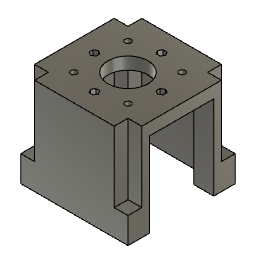
底座第三版v1 v3 (Autodesk Fusion 360 design; units mm, degrees)
Autodesk Fusion 360 part; units mm, degrees
sketch "草图1" plane through (0, 0, 0) normal (0, 0, 1) x (1, 0, 0)
  line L0 (0, 0) -> (70, 0)
  line L1 (70, 0) -> (70, 70)
  line L2 (70, 70) -> (0, 70)
  line L3 (0, 70) -> (0, 0)
  dimension "d1" = 70
  dimension "d2" = 70
  constraint horizontal L0
  constraint vertical L1
  constraint horizontal L2
  constraint vertical L3
  constraint coincident L0.start L3.end
  measures "d1" distance of L0.start L0.end
  measures "d2" distance of L0.start L2.end
extrude "拉伸1" add sketch "草图1" along normal blind 20
sketch "草图2" plane through (0, 0, 20) normal (0, 0, 1) x (-1, 0, 0)
  line L0 (0, -70) -> (0, 0)
  line L1 (0, 0) -> (-70, 0)
  line L2 (-70, 0) -> (-70, -70)
  line L3 (-70, -70) -> (0, -70)
  line L4 (-13.4, -56.6) -> (-56.6, -56.6)
  line L5 (-56.6, -56.6) -> (-56.6, -13.4)
  line L6 (-56.6, -13.4) -> (-13.4, -13.4)
  line L7 (-13.4, -13.4) -> (-13.4, -56.6)
  dimension "d5" = 43.2
  dimension "d6" = 43.2
  dimension "d7" = 13.4
  dimension "d8" = 13.4
  constraint horizontal L4
  constraint vertical L5
  constraint horizontal L6
  constraint vertical L7
  measures "d5" distance of L4.start L4.end
  measures "d6" distance of L4.start L6.end
  measures "d7" distance of L0 L7
  measures "d8" distance of L3 L4
extrude "拉伸2" cut sketch "草图2" against normal blind 6.5 contours L4 L5 L6 L7
sketch "草图3" plane through (0, 0, 13.5) normal (0, 0, 1) x (-1, 0, 0)
  line L0 (-13.4, -13.4) -> (-56.6, -13.4)
  line L1 (-56.6, -13.4) -> (-56.6, -56.6)
  line L2 (-56.6, -56.6) -> (-13.4, -56.6)
  line L3 (-13.4, -56.6) -> (-13.4, -13.4)
  circle A0 centre (-35, -35) radius 25
  line L4 (-56.6, -13.4) -> (-35, -35)
  circle A1 centre (-52.6777, -17.3223) radius 0.4987
  point P0 (-52.6777, -52.6777)
  point P1 (-17.3223, -52.6777)
  point P2 (-17.3223, -17.3223)
  dimension "d11" = 50
  dimension "d12" = 21.6
  dimension "d13" = 21.6
  dimension "d15" = 360
  constraint coincident L0.end L1.start
  constraint coincident A0.centre L4.end
  constraint coincident L4 A1.centre
  constraint coincident A0 A1.centre
  measures "d11" diameter of A0
  measures "d12" distance of L0 A0.centre
  measures "d13" distance of L1 A0.centre
hole "孔1" at (17.3223, 17.3223, 13.5) at (52.6777, 17.3223, 13.5) at (52.6777, 52.6777, 13.5) at (17.3223, 52.6777, 13.5) direction (0, 0, -1) diameter 4 end through all
sketch "草图4" plane through (0, 0, 13.5) normal (0, 0, 1) x (-1, 0, 0)
  circle A0 centre (-52.6777, -52.6777) radius 2
  circle A1 centre (-17.3223, -17.3223) radius 2
  circle A2 centre (-52.6777, -17.3223) radius 2
  circle A3 centre (-17.3223, -52.6777) radius 2
  line L0 (-13.4, -13.4) -> (-56.6, -13.4)
  line L1 (-56.6, -13.4) -> (-56.6, -56.6)
  line L2 (-56.6, -56.6) -> (-13.4, -56.6)
  line L3 (-13.4, -56.6) -> (-13.4, -13.4)
  circle A4 centre (-35, -35) radius 13.05
  dimension "d19" = 26.1
  dimension "d20" = 21.6
  dimension "d21" = 21.6
  measures "d19" diameter of A4
  measures "d20" distance of L3 A4.centre
  measures "d21" distance of L0 A4.centre
extrude "拉伸3" cut sketch "草图4" against normal blind 3.8 contours A4
sketch "草图5" plane through (0, 0, 9.7) normal (0, 0, 1) x (-1, 0, 0)
  circle A0 centre (-35, -35) radius 13.05
  circle A1 centre (-35, -35) radius 2.55
  dimension "d24" = 5.1
  constraint concentric A0 A1
  measures "d24" diameter of A1
extrude "拉伸4" cut sketch "草图5" against normal blind 100 contours A1
sketch "草图6" plane through (0, 0, 0) normal (0, 0, -1) x (1, 0, 0)
  circle A0 centre (35, -35) radius 2.55
  circle A1 centre (52.6777, -52.6777) radius 2
  circle A2 centre (17.3223, -17.3223) radius 2
  circle A3 centre (52.6777, -17.3223) radius 2
  circle A4 centre (17.3223, -52.6777) radius 2
  line L0 (0, 0) -> (0, -70)
  line L1 (0, -70) -> (70, -70)
  line L2 (70, -70) -> (70, 0)
  line L3 (70, 0) -> (0, 0)
  line L4 (35, -64.9106) -> (64.9106, -35)
  line L5 (64.9106, -35) -> (35, -5.0894)
  line L6 (35, -64.9106) -> (5.0893, -35)
  line L7 (5.0893, -35) -> (35, -5.0894)
  line L8 (64.9106, -35) -> (5.0893, -35)
  line L9 (35, -64.9106) -> (35, -5.0894)
  point P0 (35, -35)
  dimension "d27" = 42.3
  dimension "d28" = 42.3
  dimension "d29" = 42.3
  dimension "d30" = 42.3
  constraint perpendicular L4 L6
  constraint midpoint L8 P0
  constraint horizontal L4.end L6.end
  measures "d27" distance of L4.start L6.end
  measures "d28" distance of L4.start L4.end
  measures "d29" distance of L4.end L5.end
  measures "d30" distance of L5.end L6.end
extrude "拉伸5" cut sketch "草图6" against normal blind 8 contours A0 L4 L8 L9 | A0 L5 L8 L9 | A0 L7 L8 L9 | A0 L6 L8 L9
extrude "拉伸6" cut 1 faces at (25.5081, 35.775, 9.7) along direction (0, 0, -1) blind 10
sketch "草图7" plane through (0, 0, 8) normal (0, 0, -1) x (1, 0, 0)
  circle A0 centre (35, -35) radius 13.05
  line L0 (35, -64.9106) -> (64.9106, -35)
  line L1 (64.9106, -35) -> (35, -5.0894)
  line L2 (35, -5.0894) -> (5.0893, -35)
  line L3 (5.0893, -35) -> (35, -64.9106)
  circle A1 centre (35, -13.0797) radius 1.5
  circle A2 centre (56.9203, -35) radius 1.5
  circle A3 centre (35, -56.9203) radius 1.5
  circle A4 centre (13.0796, -35) radius 1.5
  dimension "d35" = 3
  dimension "d36" = 5.65
  dimension "d37" = 5.65
  dimension "d38" = 5.65
  dimension "d39" = 5.65
  dimension "d40" = 5.65
  dimension "d41" = 5.65
  dimension "d42" = 5.65
  dimension "d43" = 5.65
  constraint equal A1 A2
  constraint equal A2 A3
  constraint equal A3 A4
  measures "d35" diameter of A1
  measures "d36" distance of L1 A1.centre
  measures "d37" distance of L2 A1.centre
  measures "d38" distance of L1 A2.centre
  measures "d39" distance of L0 A2.centre
  measures "d40" distance of L0 A3.centre
  measures "d41" distance of L3 A3.centre
  measures "d42" distance of L2 A4.centre
  measures "d43" distance of L3 A4.centre
hole "孔2" at (35, 13.0797, 8) at (56.9203, 35, 8) at (13.0796, 35, 8) at (35, 56.9203, 8) direction (0, 0, 1) diameter 3 end through all
sketch "草图8" plane through (0, 0, 20) normal (0, 0, 1) x (-1, 0, 0)
  line L0 (0, -70) -> (0, 0)
  line L1 (0, 0) -> (-70, 0)
  line L2 (-70, 0) -> (-70, -70)
  line L3 (-70, -70) -> (0, -70)
  arc A0 (-13.4, -36.4654) -> (-13.4, -33.5346) centre (-13.0796, -35) ccw
  line L4 (-13.4, -36.4654) -> (-13.4, -56.6)
  line L5 (-13.4, -56.6) -> (-33.5346, -56.6)
  arc A1 (-36.4654, -56.6) -> (-33.5346, -56.6) centre (-35, -56.9203) ccw
  line L6 (-36.4654, -56.6) -> (-56.6, -56.6)
  line L7 (-56.6, -56.6) -> (-56.6, -36.4654)
  arc A2 (-56.6, -33.5346) -> (-56.6, -36.4654) centre (-56.9203, -35) ccw
  line L8 (-56.6, -33.5346) -> (-56.6, -13.4)
  line L9 (-56.6, -13.4) -> (-36.4654, -13.4)
  arc A3 (-33.5346, -13.4) -> (-36.4654, -13.4) centre (-35, -13.0797) ccw
  line L10 (-33.5346, -13.4) -> (-13.4, -13.4)
  line L11 (-13.4, -13.4) -> (-13.4, -33.5346)
  line L12 (-33.7009, -15.3297) -> (-32.4019, -13.0797)
  line L13 (-32.4019, -13.0797) -> (-33.7009, -10.8297)
  line L14 (-33.7009, -10.8297) -> (-36.299, -10.8297)
  line L15 (-36.299, -10.8297) -> (-37.598, -13.0797)
  line L16 (-37.598, -13.0797) -> (-36.299, -15.3297)
  line L17 (-36.299, -15.3297) -> (-33.7009, -15.3297)
  line L18 (-56.6, -13.4) -> (-13.4, -56.6)
  line L19 (-56.6, -56.6) -> (-13.4, -13.4)
  line L20 (-59.1703, -33.7009) -> (-59.1703, -36.299)
  line L21 (-56.9203, -32.4019) -> (-59.1703, -33.7009)
  line L22 (-54.6703, -33.7009) -> (-56.9203, -32.4019)
  line L23 (-54.6703, -36.299) -> (-54.6703, -33.7009)
  line L24 (-56.9203, -37.598) -> (-54.6703, -36.299)
  line L25 (-59.1703, -36.299) -> (-56.9203, -37.598)
  line L26 (-36.2991, -59.1703) -> (-33.701, -59.1703)
  line L27 (-37.5981, -56.9203) -> (-36.2991, -59.1703)
  line L28 (-36.2991, -54.6703) -> (-37.5981, -56.9203)
  line L29 (-33.701, -54.6703) -> (-36.2991, -54.6703)
  line L30 (-32.402, -56.9203) -> (-33.701, -54.6703)
  line L31 (-33.701, -59.1703) -> (-32.402, -56.9203)
  line L32 (-10.8297, -36.2991) -> (-10.8297, -33.701)
  line L33 (-13.0797, -37.5981) -> (-10.8297, -36.2991)
  line L34 (-15.3297, -36.2991) -> (-13.0797, -37.5981)
  line L35 (-15.3297, -33.701) -> (-15.3297, -36.2991)
  line L36 (-13.0797, -32.402) -> (-15.3297, -33.701)
  line L37 (-10.8297, -33.701) -> (-13.0797, -32.402)
  point P0 (-35, -13.0797)
  point P1 (-35, -35)
  dimension "d47" = 2.25
  dimension "d49" = 360
  constraint coincident P0 A3.centre
  constraint coincident L8.end L9.start
  constraint coincident L4.end L5.start
  constraint coincident L6.end L7.start
  constraint coincident L10.end L11.start
  constraint midpoint L19 P1
  measures "d47" distance of P0 L17
extrude "拉伸7" cut sketch "草图8" against normal blind 10 contours A0 L4 L11 L34 L35 L36 | A0 L4 L11 L32 L33 L34 L36 L37 | L5 A1 L6 L26 L27 L28 L30 L31 | L5 A1 L6 L28 L29 L30 | L9 A3 L10 L12 L16 L17 | L9 A3 L10 L12 L13 L14 L15 L16 | L7 A2 L8 L22 L23 L24 | L7 A2 L8 L20 L21 L22 L24 L25
sketch "草图9" plane through (0, 0, 0) normal (0, 0, -1) x (1, 0, 0)
  line L0 (35, -5.0894) -> (64.9106, -35)
  line L1 (64.9106, -35) -> (35, -64.9106)
  line L2 (35, -64.9106) -> (5.0893, -35)
  line L3 (5.0893, -35) -> (35, -5.0894)
  circle A0 centre (52.6777, -52.6777) radius 2
  circle A1 centre (17.3223, -17.3223) radius 2
  circle A2 centre (52.6777, -17.3223) radius 2
  circle A3 centre (17.3223, -52.6777) radius 2
  line L4 (0, 0) -> (0, -70)
  line L5 (0, -70) -> (70, -70)
  line L6 (70, -70) -> (70, 0)
  line L7 (70, 0) -> (0, 0)
extrude "拉伸8" cut sketch "草图9" against normal blind 3.5
extrude "拉伸9" cut 1 faces at (52.5592, 6.8039, 3.5) along direction (0, 0, 1) blind 4.5
sketch "草图10" plane through (0, 0, 8) normal (0, 0, -1) x (1, 0, 0)
  line L0 (70, 0) -> (0, 0)
  line L1 (0, 0) -> (0, -70)
  line L2 (0, -70) -> (70, -70)
  line L3 (70, -70) -> (70, 0)
  circle A0 centre (52.6777, -17.3223) radius 2
  circle A1 centre (52.6777, -52.6777) radius 2
  circle A2 centre (17.3223, -17.3223) radius 2
  circle A3 centre (17.3223, -52.6777) radius 2
  circle A4 centre (13.0796, -35) radius 1.5
  circle A5 centre (35, -13.0797) radius 1.5
  circle A6 centre (56.9203, -35) radius 1.5
  circle A7 centre (35, -56.9203) radius 1.5
  circle A8 centre (35, -35) radius 13.05
  line L4 (50.6569, -49.1777) -> (48.6362, -52.6777)
  line L5 (48.6362, -52.6777) -> (50.6569, -56.1777)
  line L6 (50.6569, -56.1777) -> (54.6984, -56.1777)
  line L7 (54.6984, -56.1777) -> (56.7191, -52.6777)
  line L8 (56.7191, -52.6777) -> (54.6984, -49.1777)
  line L9 (54.6984, -49.1777) -> (50.6569, -49.1777)
  line L10 (56.1777, -19.3431) -> (56.1777, -15.3016)
  line L11 (49.1777, -19.3431) -> (52.6777, -21.3638)
  line L12 (52.6777, -21.3638) -> (56.1777, -19.3431)
  line L13 (56.1777, -15.3016) -> (52.6777, -13.2809)
  line L14 (52.6777, -13.2809) -> (49.1777, -15.3016)
  line L15 (49.1777, -15.3016) -> (49.1777, -19.3431)
  line L16 (19.3431, -13.8223) -> (15.3016, -13.8223)
  line L17 (19.3431, -20.8223) -> (21.3638, -17.3223)
  line L18 (21.3638, -17.3223) -> (19.3431, -13.8223)
  line L19 (15.3016, -13.8223) -> (13.2809, -17.3223)
  line L20 (13.2809, -17.3223) -> (15.3016, -20.8223)
  line L21 (15.3016, -20.8223) -> (19.3431, -20.8223)
  line L22 (13.8223, -50.6569) -> (13.8223, -54.6984)
  line L23 (20.8223, -50.6569) -> (17.3223, -48.6362)
  line L24 (17.3223, -48.6362) -> (13.8223, -50.6569)
  line L25 (13.8223, -54.6984) -> (17.3223, -56.7191)
  line L26 (17.3223, -56.7191) -> (20.8223, -54.6984)
  line L27 (20.8223, -54.6984) -> (20.8223, -50.6569)
  point P0 (52.6777, -52.6777)
  dimension "d56" = 3.5
  dimension "d58" = 360
  constraint coincident P0 A1.centre
  measures "d56" distance of P0 L9
extrude "拉伸10" cut sketch "草图10" against normal blind 3.2 contours L4 L5 L6 L7 L8 L9 | L10 L11 L12 L13 L14 L15 | L16 L17 L18 L19 L20 L21 | L22 L23 L24 L25 L26 L27
sketch "草图12" plane through (0, 0, 8) normal (0, 0, -1) x (1, 0, 0)
  line L0 (17.3223, -48.6362) -> (20.8223, -50.6569)
  line L1 (20.8223, -50.6569) -> (20.8223, -54.6984)
  line L2 (20.8223, -54.6984) -> (17.3223, -56.7191)
  line L3 (17.3223, -56.7191) -> (13.8223, -54.6984)
  line L4 (13.8223, -54.6984) -> (13.8223, -50.6569)
  line L5 (13.8223, -50.6569) -> (17.3223, -48.6362)
  line L6 (21.3638, -17.3223) -> (19.3431, -20.8223)
  line L7 (19.3431, -20.8223) -> (15.3016, -20.8223)
  line L8 (15.3016, -20.8223) -> (13.2809, -17.3223)
  line L9 (13.2809, -17.3223) -> (15.3016, -13.8223)
  line L10 (15.3016, -13.8223) -> (19.3431, -13.8223)
  line L11 (19.3431, -13.8223) -> (21.3638, -17.3223)
  line L12 (48.6362, -52.6777) -> (50.6569, -49.1777)
  line L13 (50.6569, -49.1777) -> (54.6984, -49.1777)
  line L14 (54.6984, -49.1777) -> (56.7191, -52.6777)
  line L15 (56.7191, -52.6777) -> (54.6984, -56.1777)
  line L16 (54.6984, -56.1777) -> (50.6569, -56.1777)
  line L17 (50.6569, -56.1777) -> (48.6362, -52.6777)
  line L18 (52.6777, -21.3638) -> (49.1777, -19.3431)
  line L19 (49.1777, -19.3431) -> (49.1777, -15.3016)
  line L20 (49.1777, -15.3016) -> (52.6777, -13.2809)
  line L21 (52.6777, -13.2809) -> (56.1777, -15.3016)
  line L22 (56.1777, -15.3016) -> (56.1777, -19.3431)
  line L23 (56.1777, -19.3431) -> (52.6777, -21.3638)
  line L24 (70, 0) -> (0, 0)
  line L25 (0, 0) -> (0, -70)
  line L26 (0, -70) -> (70, -70)
  line L27 (70, -70) -> (70, 0)
  circle A0 centre (13.0796, -35) radius 1.5
  circle A1 centre (35, -13.0797) radius 1.5
  circle A2 centre (56.9203, -35) radius 1.5
  circle A3 centre (35, -56.9203) radius 1.5
  circle A4 centre (35, -35) radius 13.05
  line L28 (70, -70) -> (0, -70)
  line L29 (0, -70) -> (0, -65)
  line L30 (0, -65) -> (70, -65)
  line L31 (70, -65) -> (70, -70)
  line L32 (70, 0) -> (0, 0)
  line L33 (0, 0) -> (0, -5)
  line L34 (0, -5) -> (70, -5)
  line L35 (70, -5) -> (70, 0)
  dimension "d64" = 5
  constraint horizontal L28
  constraint vertical L29
  constraint horizontal L30
  constraint vertical L31
  constraint coincident L25 L29.end
  constraint coincident L26.end L27.start
  constraint horizontal L32
  constraint vertical L33
  constraint horizontal L34
  constraint vertical L35
  constraint coincident L25 L33.end
  constraint coincident L24.start L27.end
  measures "d64" distance of L26.end L30.end
extrude "拉伸11" add sketch "草图12" along normal blind 60 contours L24 L25 L27 L32 L33 L34 L35 | L25 L26 L27 L28 L29 L30 L31
sketch "草图13" plane through (0, 0, 8) normal (0, 0, -1) x (1, 0, 0)
  circle A0 centre (35, -35) radius 13.05
  circle A1 centre (35, -56.9203) radius 1.5
  circle A2 centre (56.9203, -35) radius 1.5
  circle A3 centre (35, -13.0797) radius 1.5
  circle A4 centre (13.0796, -35) radius 1.5
  line L0 (52.6777, -21.3638) -> (49.1777, -19.3431)
  line L1 (49.1777, -19.3431) -> (49.1777, -15.3016)
  line L2 (49.1777, -15.3016) -> (52.6777, -13.2809)
  line L3 (52.6777, -13.2809) -> (56.1777, -15.3016)
  line L4 (56.1777, -15.3016) -> (56.1777, -19.3431)
  line L5 (56.1777, -19.3431) -> (52.6777, -21.3638)
  line L6 (48.6362, -52.6777) -> (50.6569, -49.1777)
  line L7 (50.6569, -49.1777) -> (54.6984, -49.1777)
  line L8 (54.6984, -49.1777) -> (56.7191, -52.6777)
  line L9 (56.7191, -52.6777) -> (54.6984, -56.1777)
  line L10 (54.6984, -56.1777) -> (50.6569, -56.1777)
  line L11 (50.6569, -56.1777) -> (48.6362, -52.6777)
  line L12 (21.3638, -17.3223) -> (19.3431, -20.8223)
  line L13 (19.3431, -20.8223) -> (15.3016, -20.8223)
  line L14 (15.3016, -20.8223) -> (13.2809, -17.3223)
  line L15 (13.2809, -17.3223) -> (15.3016, -13.8223)
  line L16 (15.3016, -13.8223) -> (19.3431, -13.8223)
  line L17 (19.3431, -13.8223) -> (21.3638, -17.3223)
  line L18 (17.3223, -48.6362) -> (20.8223, -50.6569)
  line L19 (20.8223, -50.6569) -> (20.8223, -54.6984)
  line L20 (20.8223, -54.6984) -> (17.3223, -56.7191)
  line L21 (17.3223, -56.7191) -> (13.8223, -54.6984)
  line L22 (13.8223, -54.6984) -> (13.8223, -50.6569)
  line L23 (13.8223, -50.6569) -> (17.3223, -48.6362)
  line L24 (0, -65) -> (70, -65)
  line L25 (70, -65) -> (70, -5)
  line L26 (70, -5) -> (0, -5)
  line L27 (0, -5) -> (0, -65)
  line L28 (0, -65) -> (5, -65)
  line L29 (5, -65) -> (5, -5)
  line L30 (5, -5) -> (0, -5)
  line L31 (0, -5) -> (0, -65)
  dimension "d67" = 5
  constraint horizontal L28
  constraint vertical L29
  constraint horizontal L30
  constraint vertical L31
  constraint coincident L24.start L27.end
  measures "d67" distance of L24.start L28.end
extrude "拉伸12" add sketch "草图13" along normal blind 60 contours L24 L26 L27 L28 L29 L30 L31
sketch "草图14" plane through (0, 0, 8) normal (0, 0, -1) x (1, 0, 0)
  line L0 (5, -5) -> (5, -65)
  line L1 (5, -65) -> (70, -65)
  line L2 (70, -65) -> (70, -5)
  line L3 (70, -5) -> (5, -5)
  line L4 (17.3223, -48.6362) -> (20.8223, -50.6569)
  line L5 (20.8223, -50.6569) -> (20.8223, -54.6984)
  line L6 (20.8223, -54.6984) -> (17.3223, -56.7191)
  line L7 (17.3223, -56.7191) -> (13.8223, -54.6984)
  line L8 (13.8223, -54.6984) -> (13.8223, -50.6569)
  line L9 (13.8223, -50.6569) -> (17.3223, -48.6362)
  line L10 (21.3638, -17.3223) -> (19.3431, -20.8223)
  line L11 (19.3431, -20.8223) -> (15.3016, -20.8223)
  line L12 (15.3016, -20.8223) -> (13.2809, -17.3223)
  line L13 (13.2809, -17.3223) -> (15.3016, -13.8223)
  line L14 (15.3016, -13.8223) -> (19.3431, -13.8223)
  line L15 (19.3431, -13.8223) -> (21.3638, -17.3223)
  line L16 (48.6362, -52.6777) -> (50.6569, -49.1777)
  line L17 (50.6569, -49.1777) -> (54.6984, -49.1777)
  line L18 (54.6984, -49.1777) -> (56.7191, -52.6777)
  line L19 (56.7191, -52.6777) -> (54.6984, -56.1777)
  line L20 (54.6984, -56.1777) -> (50.6569, -56.1777)
  line L21 (50.6569, -56.1777) -> (48.6362, -52.6777)
  line L22 (52.6777, -21.3638) -> (49.1777, -19.3431)
  line L23 (49.1777, -19.3431) -> (49.1777, -15.3016)
  line L24 (49.1777, -15.3016) -> (52.6777, -13.2809)
  line L25 (52.6777, -13.2809) -> (56.1777, -15.3016)
  line L26 (56.1777, -15.3016) -> (56.1777, -19.3431)
  line L27 (56.1777, -19.3431) -> (52.6777, -21.3638)
  circle A0 centre (13.0796, -35) radius 1.5
  circle A1 centre (35, -13.0797) radius 1.5
  circle A2 centre (56.9203, -35) radius 1.5
  circle A3 centre (35, -56.9203) radius 1.5
  circle A4 centre (35, -35) radius 13.05
  line L28 (70, -5) -> (61, -5)
  line L29 (61, -5) -> (61, -14)
  line L30 (61, -14) -> (70, -14)
  line L31 (70, -14) -> (70, -5)
  line L32 (5, -5) -> (14, -5)
  line L33 (14, -5) -> (14, -14)
  line L34 (14, -14) -> (5, -14)
  line L35 (5, -14) -> (5, -5)
  line L36 (5, -65) -> (14, -65)
  line L37 (14, -65) -> (14, -56)
  line L38 (14, -56) -> (5, -56)
  line L39 (5, -56) -> (5, -65)
  line L40 (70, -65) -> (61, -65)
  line L41 (61, -65) -> (61, -56)
  line L42 (61, -56) -> (70, -56)
  line L43 (70, -56) -> (70, -65)
  dimension "d70" = 9
  dimension "d71" = 9
  dimension "d72" = 9
  dimension "d73" = 9
  dimension "d74" = 9
  dimension "d75" = 9
  dimension "d76" = 9
  dimension "d77" = 9
  constraint horizontal L28
  constraint vertical L29
  constraint horizontal L30
  constraint vertical L31
  constraint coincident L2.end L3.start
  constraint horizontal L32
  constraint vertical L33
  constraint horizontal L34
  constraint vertical L35
  constraint coincident L0.start L3.end
  constraint horizontal L36
  constraint vertical L37
  constraint horizontal L38
  constraint vertical L39
  constraint coincident L0.end L1.start
  constraint horizontal L40
  constraint vertical L41
  constraint horizontal L42
  constraint vertical L43
  constraint coincident L1.end L2.start
  measures "d70" distance of L2.end L28.end
  measures "d71" distance of L2.end L30.end
  measures "d72" distance of L0.start L32.end
  measures "d73" distance of L0.start L34.end
  measures "d74" distance of L0.end L36.end
  measures "d75" distance of L0.end L38.end
  measures "d76" distance of L1.end L40.end
  measures "d77" distance of L1.end L42.end
extrude "拉伸13" add sketch "草图14" along normal blind 60 contours L0 L3 L32 L33 L34 L35 | L0 L1 L36 L37 L38 L39 | L2 L3 L28 L29 L30 L31 | L1 L2 L40 L41 L42 L43
sketch "草图15" plane through (0, 0, 8) normal (0, 0, -1) x (1, 0, 0)
  line L0 (17.3223, -48.6362) -> (20.8223, -50.6569)
  line L1 (20.8223, -50.6569) -> (20.8223, -54.6984)
  line L2 (20.8223, -54.6984) -> (17.3223, -56.7191)
  line L3 (17.3223, -56.7191) -> (13.8223, -54.6984)
  line L4 (13.8223, -54.6984) -> (13.8223, -50.6569)
  line L5 (13.8223, -50.6569) -> (17.3223, -48.6362)
  line L6 (21.3638, -17.3223) -> (19.3431, -20.8223)
  line L7 (19.3431, -20.8223) -> (15.3016, -20.8223)
  line L8 (15.3016, -20.8223) -> (13.2809, -17.3223)
  line L9 (13.2809, -17.3223) -> (15.3016, -13.8223)
  line L10 (15.3016, -13.8223) -> (19.3431, -13.8223)
  line L11 (19.3431, -13.8223) -> (21.3638, -17.3223)
  line L12 (48.6362, -52.6777) -> (50.6569, -49.1777)
  line L13 (50.6569, -49.1777) -> (54.6984, -49.1777)
  line L14 (54.6984, -49.1777) -> (56.7191, -52.6777)
  line L15 (56.7191, -52.6777) -> (54.6984, -56.1777)
  line L16 (54.6984, -56.1777) -> (50.6569, -56.1777)
  line L17 (50.6569, -56.1777) -> (48.6362, -52.6777)
  line L18 (52.6777, -21.3638) -> (49.1777, -19.3431)
  line L19 (49.1777, -19.3431) -> (49.1777, -15.3016)
  line L20 (49.1777, -15.3016) -> (52.6777, -13.2809)
  line L21 (52.6777, -13.2809) -> (56.1777, -15.3016)
  line L22 (56.1777, -15.3016) -> (56.1777, -19.3431)
  line L23 (56.1777, -19.3431) -> (52.6777, -21.3638)
  circle A0 centre (13.0796, -35) radius 1.5
  circle A1 centre (35, -13.0797) radius 1.5
  circle A2 centre (56.9203, -35) radius 1.5
  circle A3 centre (35, -56.9203) radius 1.5
  circle A4 centre (35, -35) radius 13.05
  line L24 (61, -65) -> (61, -56)
  line L25 (61, -56) -> (70, -56)
  line L26 (70, -56) -> (70, -14)
  line L27 (70, -14) -> (61, -14)
  line L28 (61, -14) -> (61, -5)
  line L29 (61, -5) -> (14, -5)
  line L30 (14, -5) -> (14, -14)
  line L31 (14, -14) -> (5, -14)
  line L32 (5, -14) -> (5, -56)
  line L33 (5, -56) -> (14, -56)
  line L34 (14, -56) -> (14, -65)
  line L35 (14, -65) -> (61, -65)
  line L36 (61, -14) -> (57, -14)
  line L37 (57, -14) -> (57, -5)
  line L38 (57, -5) -> (61, -5)
  line L39 (61, -5) -> (61, -14)
  line L40 (61, -56) -> (57, -56)
  line L41 (57, -56) -> (57, -65)
  line L42 (57, -65) -> (61, -65)
  line L43 (61, -65) -> (61, -56)
  dimension "d80" = 4
  dimension "d81" = 4
  constraint horizontal L36
  constraint vertical L37
  constraint horizontal L38
  constraint vertical L39
  constraint coincident L27.end L28.start
  constraint horizontal L40
  constraint vertical L41
  constraint horizontal L42
  constraint vertical L43
  constraint coincident L24.end L25.start
  measures "d80" distance of L27.end L36.end
  measures "d81" distance of L24.end L40.end
extrude "拉伸14" add sketch "草图15" along normal blind 60 contours L24 L35 L40 L41 L42 L43 | L28 L29 L36 L37 L38 L39
sketch "草图16" plane through (0, 0, 20) normal (0, 0, 1) x (-1, 0, 0)
  line L0 (-56.9203, -32.4019) -> (-56.6, -32.5868)
  line L1 (-56.6, -32.5868) -> (-56.6, -13.4)
  line L2 (-56.6, -13.4) -> (-37.4131, -13.4)
  line L3 (-37.4131, -13.4) -> (-37.598, -13.0797)
  line L4 (-37.598, -13.0797) -> (-36.299, -10.8297)
  line L5 (-36.299, -10.8297) -> (-33.7009, -10.8297)
  line L6 (-33.7009, -10.8297) -> (-32.4019, -13.0797)
  line L7 (-32.4019, -13.0797) -> (-32.5868, -13.4)
  line L8 (-32.5868, -13.4) -> (-13.4, -13.4)
  line L9 (-13.4, -13.4) -> (-13.4, -32.5869)
  line L10 (-13.4, -32.5869) -> (-13.0797, -32.402)
  line L11 (-13.0797, -32.402) -> (-10.8297, -33.701)
  line L12 (-10.8297, -33.701) -> (-10.8297, -36.2991)
  line L13 (-10.8297, -36.2991) -> (-13.0797, -37.5981)
  line L14 (-13.0797, -37.5981) -> (-13.4, -37.4132)
  line L15 (-13.4, -37.4132) -> (-13.4, -56.6)
  line L16 (-13.4, -56.6) -> (-32.5869, -56.6)
  line L17 (-32.5869, -56.6) -> (-32.402, -56.9203)
  line L18 (-32.402, -56.9203) -> (-33.701, -59.1703)
  line L19 (-33.701, -59.1703) -> (-36.2991, -59.1703)
  line L20 (-36.2991, -59.1703) -> (-37.5981, -56.9203)
  line L21 (-37.5981, -56.9203) -> (-37.4132, -56.6)
  line L22 (-37.4132, -56.6) -> (-56.6, -56.6)
  line L23 (-56.6, -56.6) -> (-56.6, -37.4131)
  line L24 (-56.6, -37.4131) -> (-56.9203, -37.598)
  line L25 (-56.9203, -37.598) -> (-59.1703, -36.299)
  line L26 (-59.1703, -36.299) -> (-59.1703, -33.7009)
  line L27 (-59.1703, -33.7009) -> (-56.9203, -32.4019)
  line L28 (0, -70) -> (0, 0)
  line L29 (0, 0) -> (-70, 0)
  line L30 (-70, 0) -> (-70, -70)
  line L31 (-70, -70) -> (0, -70)
  line L32 (0, -70) -> (-9, -70)
  line L33 (-9, -70) -> (-9, -61)
  line L34 (-9, -61) -> (0, -61)
  line L35 (0, -61) -> (0, -70)
  line L36 (-70, -70) -> (-61, -70)
  line L37 (-61, -70) -> (-61, -61)
  line L38 (-61, -61) -> (-70, -61)
  line L39 (-70, -61) -> (-70, -70)
  line L40 (-70, 0) -> (-61, 0)
  line L41 (-61, 0) -> (-61, -9)
  line L42 (-61, -9) -> (-70, -9)
  line L43 (-70, -9) -> (-70, 0)
  line L44 (0, 0) -> (-9, 0)
  line L45 (-9, 0) -> (-9, -9)
  line L46 (-9, -9) -> (0, -9)
  line L47 (0, -9) -> (0, 0)
  dimension "d84" = 9
  dimension "d85" = 9
  dimension "d86" = 9
  dimension "d87" = 9
  dimension "d88" = 9
  dimension "d89" = 9
  dimension "d90" = 9
  dimension "d91" = 9
  constraint horizontal L32
  constraint vertical L33
  constraint horizontal L34
  constraint vertical L35
  constraint coincident L28.start L31.end
  constraint horizontal L36
  constraint vertical L37
  constraint horizontal L38
  constraint vertical L39
  constraint coincident L30.end L31.start
  constraint horizontal L40
  constraint vertical L41
  constraint horizontal L42
  constraint vertical L43
  constraint coincident L29.end L30.start
  constraint horizontal L44
  constraint vertical L45
  constraint horizontal L46
  constraint vertical L47
  constraint coincident L28.end L29.start
  measures "d84" distance of L28.start L32.end
  measures "d85" distance of L28.start L34.end
  measures "d86" distance of L30.end L36.end
  measures "d87" distance of L30.end L38.end
  measures "d88" distance of L29.end L40.end
  measures "d89" distance of L29.end L42.end
  measures "d90" distance of L28.end L44.end
  measures "d91" distance of L28.end L46.end
extrude "拉伸15" cut sketch "草图16" against normal blind 50 contours L28 L31 L32 L33 L34 L35 | L28 L29 L44 L45 L46 L47 | L30 L31 L36 L37 L38 L39 | L29 L30 L40 L41 L42 L43
extrude "拉伸16" cut 1 faces at (65.6667, 6.3333, -52) along direction (0, 0, 1) blind 10
extrude "拉伸17" cut 1 faces at (3.6099, 34.567, 20) along direction (0, 0, -1) blind 6.5
extrude "拉伸18" add 1 faces at (3.6099, 34.567, 13.5) along direction (0, 0, 1) blind 2.5
extrude "拉伸19" add 1 faces at (65.6667, 6.3333, -42) along direction (0, 0, -1) blind 5
